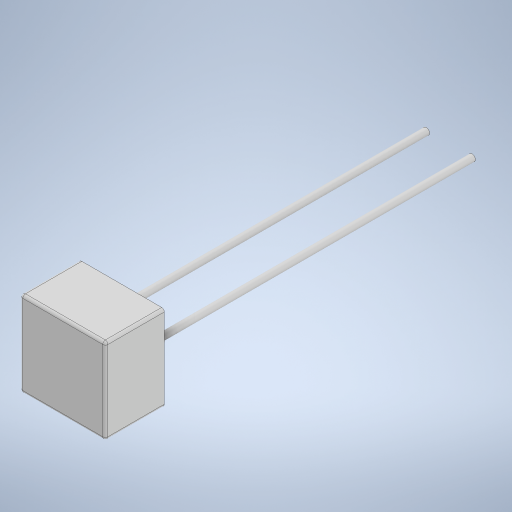
# Autodesk Inventor part: KM6A-M1500
Saved by Autodesk Inventor 2024 (Build 280153000, 153)
## iProperties
Created: 2023-12-19
Part Number: KM6A-M1500
Material: Generic
Document SubType Name: Sheet Metal
Designer: user
Density: 1 g/cm^3
Sheet Metal Rule: Default
Appearance: Default
Author: user
Autodesk Inventor part; units mm, degrees
sketch "Sketch1" plane through (0, 0, 0) normal (0, 0, 1) x (1, 0, 0)
  line L0 (0.2, 0) -> (6.3, 0)
  line L1 (6.5, 0.2) -> (6.5, 6.3)
  line L2 (6.3, 6.5) -> (0.2, 6.5)
  line L3 (0, 6.3) -> (0, 0.2)
  arc A0 (0.2, 6.5) -> (0, 6.3) centre (0.2, 6.3) ccw
  arc A1 (6.5, 6.3) -> (6.3, 6.5) centre (6.3, 6.3) ccw
  arc A2 (6.3, 0) -> (6.5, 0.2) centre (6.3, 0.2) ccw
  arc A3 (0, 0.2) -> (0.2, 0) centre (0.2, 0.2) ccw
  point P0 (0, 0)
  point P1 (6.5, 6.5)
  point P2 (6.5, 0)
  point P3 (0, 6.5)
  dimension "d0" = 6.5
  dimension "d1" = 6.5
  dimension "d2" = 0.2
  constraints: 8 end point, 8 point on circle, 8 point on line, 8 tangent, 4 centre point, 3 equal radius, 2 parallel, 1 horizontal, 1 perpendicular
  measures "d0" distance of point (0, 6.5) point (6.5, 6.5)
  measures "d1" distance of point (6.5, 6.5) point (6.5, 0)
  measures "d2" radius of A0
extrude "Extrusion1" add sketch "Sketch1" along normal mid plane 4.5
fillet "Fillet1" radius 0.2 8 edges at (0.0586, 0.0586, 2.25) (3.25, 0, 2.25) (6.4414, 0.0586, 2.25) (6.5, 3.25, 2.25) (6.4414, 6.4414, 2.25) (3.25, 6.5, 2.25) (0.0586, 6.4414, 2.25) (0, 3.25, 2.25)
ref_plane "Work Plane1" through (0.2, 3.25, -2.25) normal (0, 1, 0) x (1, 0, 0)
sketch "Sketch2" plane through (0.2, 3.25, -2.25) normal (0, 1, 0) x (1, 0, 0)
  line L0 (1.3, 0) -> (1.3, 25)
  line L1 (4.8, 0) -> (4.8, 25)
  point P0 (-0.2, -2.25)
  point P1 (-0.2, 0)
  point P2 (6.3, 0)
  dimension "d6" = 1.5
  dimension "d7" = 1.5
  dimension "d8" = 25
  dimension "d9" = 25
  constraints: 4 end point, 2 vertical
  measures "d6" distance of point (-0.2, 0) L0.start
  measures "d7" distance of point (6.3, 0) L1.start
  measures "d8" distance of L0.start L0.end
  measures "d9" distance of L1.start L1.end
sketch "Sketch3" plane through (0, 0, -2.25) normal (0, 0, -1) x (-1, 0, 0)
  circle A0 centre (-1.5017, 3.2491) radius 0.4
  circle A1 centre (-5.0012, 3.2491) radius 0.4
  point P0 (0, 0)
  dimension "d10" = 0.8
  dimension "d11" = 0.8
  constraints: 2 centre point
  measures "d10" diameter of A0
  measures "d11" diameter of A1
extrude "Extrusion2" add sketch "Sketch3" along normal blind 1.25 contours A0
extrude "Extrusion3" add sketch "Sketch3" along normal blind 1.25 contours A1
fillet "Fillet2" radius 0.2 2 edges at (1.9017, 3.2491, -3.5) (5.4012, 3.2491, -3.5)
ref_plane "Work Plane2" through (1.5017, 3.2491, -3.5) normal (0, 0, -1) x (-1, 0, 0)
ref_plane "Work Plane3" through (5.0012, 3.2491, -3.5) normal (0, 0, -1) x (-1, 0, 0)
sketch "Sketch4" plane through (1.5017, 3.2491, -3.5) normal (0, 0, -1) x (-1, 0, 0)
  circle A0 centre (0, 0) radius 0.25
  point P0 (1.5017, -3.2491)
  dimension "d19" = 0.5
  constraints: 1 centre point
  measures "d19" diameter of A0
sketch "Sketch5" plane through (5.0012, 3.2491, -3.5) normal (0, 0, -1) x (-1, 0, 0)
  circle A0 centre (0, 0) radius 0.25
  point P0 (5.0012, -3.2491)
  dimension "d20" = 0.5
  constraints: 1 centre point
  measures "d20" diameter of A0
sweep "Sweep1" add profiles "Sketch4" path "Sketch2" path curves L0
sweep "Sweep2" add profiles "Sketch5" path "Sketch2" path curves L1
equation "\"BendRadius\" = Thickness"
equation "\"BendReliefWidth\" = Thickness"
equation "\"BendReliefDepth\" = 0.5 * Thickness"
equation "\"CornerReliefSize\" = 4 * Thickness"
equation "\"MinimumRemnant\" = 2 * Thickness"
equation "\"TransitionRadius\" = BendRadius"
equation "\"JacobiRadiusSize\" = BendRadius"
equation "\"GapSize\" = Thickness"
equation "\"Thickness\" = 3.048"
body "Solid1"
